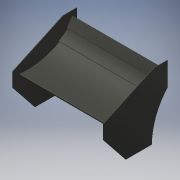
# Autodesk Inventor part: R-wing
Saved by Autodesk Inventor 2018.1 (Build 221171000, 171)
## iProperties
Created: 2017-10-11
Part Number: R-wing
Material: CFRP
Document SubType Name: Modeling
Designer: kuwano
Density: 1.43 g/cm^3
Appearance: カーボンファイバー 1
Mass: 3862.06 g
Surface Area: 54014.8 cm^2
Volume: 2700.74 cm^3
Author: kuwano
Autodesk Inventor part; units mm, degrees
ref_plane "YZ Plane" through (0, 0, 0) normal (1, 0, 0) x (0, 1, 0)
ref_plane "XZ Plane" through (0, 0, 0) normal (0, 1, 0) x (-1, 0, 0)
ref_plane "XY Plane" through (0, 0, 0) normal (0, 0, 1) x (1, 0, 0)
sketch "スケッチ1" plane through (0, 0, 0) normal (1, 0, 0) x (0, 1, 0)
  arc A0 (0, 250) -> (88.1635, -250) centre (324.5919, 49.4615) ccw
  line L0 (0, 250) -> (88.1635, -250)
  line L1 (0, -524.7592) -> (0, 478.123) projected
  line L2 (-256.4277, 0) -> (871.9069, 0) projected
  arc A1 (72.5067, -190) -> (177.5379, -340) centre (323.9512, -125.7085) ccw
  line L3 (72.5067, -190) -> (177.5379, -340)
  arc A2 (148.6314, -290) -> (262.8832, -370) centre (671.2931, 334.8541) ccw
  arc A3 (148.6314, -290) -> (262.8832, -370) centre (301.1676, -193.74) ccw
  line L4 (148.6314, -290) -> (262.8832, -370)
  arc A4 (0, 250) -> (88.1635, -250) centre (710.7162, 117.5456) ccw
  arc A5 (72.5067, -190) -> (177.5379, -340) centre (644.3089, 98.6084) ccw
  dimension "d14" = 10
  dimension "d15" = 250
  dimension "d18" = 25
  dimension "d19" = 60
  dimension "d20" = 150
  dimension "d21" = 500
  dimension "d22" = 20
  dimension "d23" = 50
  dimension "d25" = 5
  dimension "d26" = 80
  dimension "d70" = 5
  constraints: 12 point on circle, 6 centre point, 6 end point, 1 point on line
  measures "d14" angle of L1 L0
  measures "d15" distance from line of L2 L0.start
  measures "d18" angle of L3 L0
  measures "d19" vertical distance of L0.end L3.start
  measures "d20" vertical distance of L3.start L3.end
  measures "d21" vertical distance of L0.end L0.start
  measures "d22" angle of L4 L3
  measures "d23" vertical distance of L3.end L4.start
  measures "d25" distance from line of L3 L4.start
  measures "d26" vertical distance of L4.end L4.start
  measures "d70" distance from line of L0 L3.start
extrude "押し出し8" add sketch "スケッチ1" along normal mid plane 970 contours A4 L2 A0 | L2 A4 L1 A0 | L1 A4 A0 | A5 A1 L0 | L0 A1 A5 | A2 A3
fillet "フィレット4" radius 10 1 edges at (0, 0, 250)
fillet "フィレット5" radius 2 3 edges at (0, 88.1635, -250) (0, 177.5379, -340) (0, 262.8832, -370)
fillet "フィレット6" radius 3 2 edges at (0, 148.6314, -290) (0, 72.5067, -190)
sketch "スケッチ6" plane through (485, 0, 0) normal (1, 0, 0) x (0, 0, -1)
  line L0 (-275.4848, -100.9038) -> (-275.4848, 50)
  line L1 (-275.4848, 50) -> (264.5152, 299.0962)
  line L2 (264.5152, 299.0962) -> (414.5152, 299.0962)
  line L3 (414.5152, 299.0962) -> (414.5152, 49.0962)
  arc A0 (414.5152, 49.0962) -> (244.5152, -400.9038) centre (925.1034, -400.9038) ccw
  line L4 (244.5152, -400.9038) -> (-35.4848, -400.9038)
  line L5 (-35.4848, -400.9038) -> (-275.4848, -100.9038)
  arc A1 (366.43, 249.0962) -> (362.8024, 250.7061) centre (364.5152, 249.6735) ccw projected
  point P0 (0, 0)
  dimension "d71" = 50
  dimension "d72" = 50
  dimension "d73" = 150
  dimension "d74" = 50
  dimension "d75" = 240
  dimension "d76" = 690
  dimension "d77" = 700
  dimension "d78" = 250
  dimension "d79" = 300
  dimension "d80" = 280
  constraints: 12 end point, 2 perpendicular, 2 point on circle, 1 centre point, 1 horizontal, 1 line through centre, 1 vertical
  measures "d71" distance from line of L3 A1.centre
  measures "d72" distance from line of A1.start L2
  measures "d73" distance from line of L3 L1.end
  measures "d74" vertical distance of point (0, 0) L0.end
  measures "d75" distance from line of L4.end L0
  measures "d76" distance between parallel lines of L3 L0
  measures "d77" distance between parallel lines of L4 L2
  measures "d78" distance of L2.end L3.end
  measures "d79" distance from line of L4 L0.start
  measures "d80" distance of L4.start L4.end
extrude "押し出し9" add sketch "スケッチ6" along normal blind 5
mirror "ミラー5" about plane through (0, 0, 0) normal (1, 0, 0) of "押し出し9"
shell "シェル1" thickness 1 removed faces 0
